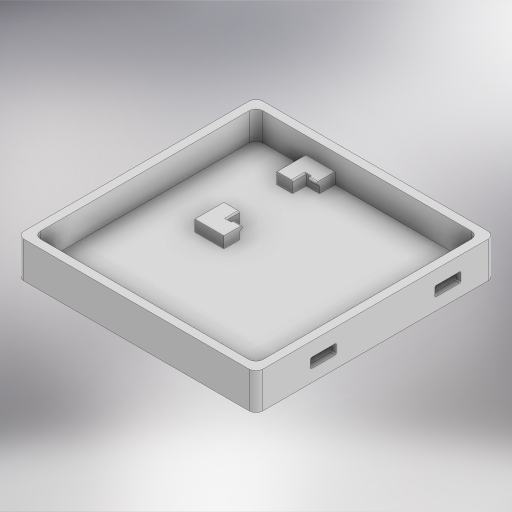
# Autodesk Inventor part: Bottom Plate
Saved by Autodesk Inventor 2024 (Build 280153000, 153)
## iProperties
Created: 2026-05-15
Part Number: Bottom Plate
Material: Generic
Document SubType Name: Modeling
Designer: Satyajit
Density: 1 g/cm^3
Appearance: Default
Author: Satyajit
Autodesk Inventor part; units mm, degrees
ref_plane "YZ Plane" through (0, 0, 0) normal (1, 0, 0) x (0, 1, 0)
ref_plane "XZ Plane" through (0, 0, 0) normal (0, 1, 0) x (-1, 0, 0)
ref_plane "XY Plane" through (0, 0, 0) normal (0, 0, 1) x (1, 0, 0)
sketch "Sketch1" plane through (0, 0, 0) normal (0, 1, 0) x (-1, 0, 0)
  line L0 (40, -40) -> (-40, -40)
  line L1 (-40, -40) -> (-40, 40)
  line L2 (-40, 40) -> (40, 40)
  line L3 (40, 40) -> (40, -40)
  line L4 (40, -40) -> (-40, 40) construction
  line L5 (-40, -40) -> (40, 40) construction
  line L6 (-43, 43) -> (-43, -43)
  line L7 (-43, -43) -> (43, -43)
  line L8 (43, -43) -> (43, 43)
  line L9 (43, 43) -> (-43, 43)
  point P0 (0, 0)
  dimension "d0" = 80
  dimension "d1" = 3
  constraints: 20 end point, 4 parallel, 3 perpendicular, 2 midpoint, 1 horizontal, 3 other
  measures "d0" distance of L1.end L2.end
  measures "d1" distance between parallel lines of L1 L6
extrude "Extrusion1" add sketch "Sketch1" against normal blind 3 contours L0 L1 L2 L3 | L9 L8 L7 L6
extrude "Extrusion2" add sketch "Sketch1" along normal blind 10
sketch "Sketch2" plane through (0, 0, 0) normal (0, 1, 0) x (1, 0, 0)
  line L0 (-16, 34) -> (41, 34)
  line L1 (41, 34) -> (41, 6)
  line L2 (41, 6) -> (-16, 6)
  line L3 (-16, 6) -> (-16, 34) construction
  line L4 (-16, 34) -> (41, 6) construction
  line L5 (41, 34) -> (-16, 6) construction
  line L6 (-16, 29.15) -> (-22, 29.15) construction
  line L7 (-22, 29.15) -> (-22, 10.85) construction
  line L8 (-22, 10.85) -> (-16, 10.85) construction
  line L9 (40, 40) -> (40, -40) projected
  line L10 (-40, -40) -> (-40, 40) construction
  line L11 (43, 43) -> (43, -43) projected
  line L12 (-40, 40) -> (40, 40) projected
  line L13 (-16.4, 29.55) -> (-16.4, 34.4)
  line L14 (-16.4, 34.4) -> (-11.55, 34.4)
  line L15 (-11.55, 34.4) -> (-11.55, 40)
  line L16 (-16.4, 29.55) -> (-22, 29.55)
  line L17 (-22, 29.55) -> (-22, 40)
  line L18 (12.5, 20) -> (-22, 20) construction
  line L19 (-16.4, 10.45) -> (-16.4, 5.6)
  line L20 (-16.4, 5.6) -> (-11.55, 5.6)
  line L21 (-11.55, 5.6) -> (-11.55, 0)
  line L22 (-16.4, 10.45) -> (-22, 10.45)
  line L23 (-22, 10.45) -> (-22, 0)
  line L24 (-22, 0) -> (-11.55, 0)
  line L25 (40, 5.5) -> (41, 5.5)
  line L26 (41, 5.5) -> (41, 6)
  line L27 (40, 34) -> (40, 34.5)
  line L28 (40, 34.5) -> (41, 34.5)
  line L29 (41, 34.5) -> (41, 34)
  point P0 (0, 0)
  point P1 (40, 6)
  dimension "d16" = 57
  dimension "d17" = 28
  dimension "d18" = 6
  dimension "d19" = 18.3
  dimension "d26" = 2
  dimension "d27" = 6
  dimension "d28" = 0.4
  dimension "d29" = 0.4
  dimension "d30" = 0.4
  dimension "d35" = 0.5
  constraints: 52 end point, 11 perpendicular, 8 point on line, 6 symmetric about line, 4 horizontal, 3 midpoint, 2 collinear, 2 parallel, 1 horizontal alignment, 1 vertical, 1 other
  measures "d16" distance of L0.start L0.end
  measures "d17" distance of L0.end L1.end
  measures "d18" distance between parallel lines of L3 L7
  measures "d19" distance of L6.end L7.end
  measures "d26" distance between parallel lines of L11 L1
  measures "d27" distance between parallel lines of L12 L0
  measures "d28" distance between parallel lines of L6 L16
  measures "d29" distance between parallel lines of L13 L3
  measures "d30" distance between parallel lines of L14 L0
  measures "d35" distance of L28.end L0.end
extrude "Extrusion3" add sketch "Sketch2" along normal blind 4 contours L12 L15 L14 L13 L16 L17 | L19 L20 L21 L24 L23 L22
extrude "Extrusion4" cut sketch "Sketch2" along normal blind 6 contours L9 L28 L29 L0 | L0 L1 L2 L9 | L2 L26 L25 L9
sketch "Sketch3" plane through (41, 0, -34.5) normal (-1, 0, 0) x (0, 0, 1)
  line L0 (29, 0) -> (0, 0) projected
  line L1 (29, 0) -> (29, 6) projected
  line L2 (29, 6) -> (0, 6) projected
  line L3 (0, 0) -> (0, 6) projected
  line L4 (4.35, 1.45) -> (12.65, 1.45)
  line L5 (13.15, 1.95) -> (13.15, 4.45)
  line L6 (12.65, 4.95) -> (4.35, 4.95)
  line L7 (3.85, 4.45) -> (3.85, 1.95)
  line L8 (3.85, 1.45) -> (13.15, 4.95) construction
  line L9 (13.15, 1.45) -> (3.85, 4.95) construction
  line L10 (14.5, 0) -> (14.5, 6) construction
  line L11 (24.65, 1.45) -> (16.35, 1.45)
  line L12 (15.85, 1.95) -> (15.85, 4.45)
  line L13 (16.35, 4.95) -> (24.65, 4.95)
  line L14 (25.15, 4.45) -> (25.15, 1.95)
  line L15 (25.15, 1.45) -> (15.85, 4.95) construction
  line L16 (15.85, 1.45) -> (25.15, 4.95) construction
  arc A0 (3.85, 1.95) -> (4.35, 1.45) centre (4.35, 1.95) ccw
  arc A1 (4.35, 4.95) -> (3.85, 4.45) centre (4.35, 4.45) ccw
  arc A2 (13.15, 4.45) -> (12.65, 4.95) centre (12.65, 4.45) ccw
  arc A3 (12.65, 1.45) -> (13.15, 1.95) centre (12.65, 1.95) ccw
  arc A4 (15.85, 1.95) -> (16.35, 1.45) centre (16.35, 1.95) ccw
  arc A5 (16.35, 4.95) -> (15.85, 4.45) centre (16.35, 4.45) ccw
  arc A6 (25.15, 4.45) -> (24.65, 4.95) centre (24.65, 4.45) ccw
  arc A7 (24.65, 1.45) -> (25.15, 1.95) centre (24.65, 1.95) ccw
  line L17 (49.1, 1.45) -> (57.4, 1.45)
  line L18 (57.9, 1.95) -> (57.9, 4.45)
  line L19 (57.4, 4.95) -> (49.1, 4.95)
  line L20 (48.6, 4.45) -> (48.6, 1.95)
  line L21 (48.6, 1.45) -> (57.9, 4.95) construction
  line L22 (57.9, 1.45) -> (48.6, 4.95) construction
  arc A8 (48.6, 1.95) -> (49.1, 1.45) centre (49.1, 1.95) ccw
  arc A9 (49.1, 4.95) -> (48.6, 4.45) centre (49.1, 4.45) ccw
  arc A10 (57.9, 4.45) -> (57.4, 4.95) centre (57.4, 4.45) ccw
  arc A11 (57.4, 1.45) -> (57.9, 1.95) centre (57.4, 1.95) ccw
  line L23 (29, 0) -> (77.5, 0)
  line L24 (77.5, -3) -> (77.5, 10) projected
  line L25 (47.25, 0) -> (47.25, 6)
  line L26 (47.25, 6) -> (59.25, 6)
  line L27 (59.25, 6) -> (59.25, 0)
  point P0 (34.5, 0)
  point P1 (8.5, 3.2)
  point P2 (20.5, 3.2)
  point P3 (20.5, 3.2)
  point P4 (53.25, 3.2)
  point P5 (53.25, 0)
  point P6 (53.25, 6)
  dimension "d36" = 9.3
  dimension "d37" = 3.5
  dimension "d40" = 12
  dimension "d41" = 3.2
  dimension "d42" = 0.5
  dimension "d45" = 9.3
  dimension "d46" = 3.5
  dimension "d47" = 0.5
  dimension "d48" = 12
  constraints: 46 end point, 27 point on line, 24 point on circle, 24 tangent, 12 centre point, 10 equal radius, 9 midpoint, 5 parallel, 5 symmetric about line, 4 perpendicular, 3 horizontal, 2 vertical alignment, 1 horizontal alignment, 1 vertical
  measures "d36" distance of L8.end L9.end
  measures "d37" distance of L9.start L8.end
  measures "d40" distance of point (8.5, 3.2) point (20.5, 3.2)
  measures "d41" distance from line of L0 point (8.5, 3.2)
  measures "d42" radius of A0
  measures "d45" distance of L21.end L22.end
  measures "d46" distance of L22.start L21.end
  measures "d47" radius of A8
  measures "d48" distance between parallel lines of L27 L25
extrude "Extrusion5" cut sketch "Sketch3" against normal blind 6 contours A0 L7 A1 L6 A2 L5 A3 L4 | A8 L20 A9 L19 A10 L18 A11 L17
extrude "Extrusion6" cut sketch "Sketch3" along normal blind 6 contours A8 L20 A9 L19 A10 L18 A11 L17 | L25 L26 L27 L23
sketch "Sketch4" plane through (0, 4, 0) normal (0, 1, 0) x (1, 0, 0)
  line L0 (-11.55, 5.6) -> (-16.4, 5.6) projected
  line L1 (-16.4, 5.6) -> (-16.4, 10.45) projected
  line L2 (-11.55, 0) -> (-11.55, 5.6) projected
  line L3 (-11.55, 5.6) -> (-11.55, 6.6)
  line L4 (-11.55, 6.6) -> (-14.55, 6.6)
  line L5 (-14.55, 6.6) -> (-14.55, 5.6)
  line L6 (-16.4, 10.45) -> (-22, 10.45) projected
  line L7 (-22, 40) -> (-22, 29.55) projected
  line L8 (-22, 10.45) -> (-22, 29.55) construction
  line L9 (-22, 20) -> (0, 20) construction
  line L10 (-22, 29.55) -> (-16.4, 29.55) projected
  line L11 (-16.4, 29.55) -> (-16.4, 34.4) projected
  line L12 (-16.4, 34.4) -> (-11.55, 34.4) projected
  line L13 (-11.55, 34.4) -> (-11.55, 33.4)
  line L14 (-11.55, 33.4) -> (-14.55, 33.4)
  line L15 (-14.55, 33.4) -> (-14.55, 34.4)
  point P0 (0, 0)
  dimension "d51" = 1
  dimension "d52" = 3
  constraints: 16 end point, 3 symmetric about line, 2 perpendicular, 2 vertical, 1 horizontal, 1 midpoint, 1 point on line, 1 vertical alignment
  measures "d51" distance of L0.start L3.end
  measures "d52" distance of L3.end L4.end
extrude "Extrusion7" add sketch "Sketch4" against normal blind 1
fillet "Fillet1" radius 0.5 4 edges at (-13.05, 4, -6.6) (-13.05, 3, -6.6) (-13.05, 4, -33.4) (-13.05, 3, -33.4)
fillet "Fillet2" radius 1 2 edges at (-13.05, 3, -5.6) (-13.05, 3, -34.4)
fillet "Fillet3" radius 0.5 24 edges at (-16.4, 4, -31.975) (-16.4, 4, -8.025) (41, 1.5964, -30.5036) (41, 3.2, -30.65) (41, 4.8036, -30.5036) (41, 4.95, -26) (41, 4.8036, -21.4964) (41, 3.2, -21.35) (41, 1.5964, -21.4964) (41, 1.45, -26) (40, 3, -34.5) (40, 6, -20) (40, 3, -5.5) (41, 1.5964, 23.2536) (41, 3.2, 23.4) (41, 4.8036, 23.2536) (41, 4.95, 18.75) (41, 4.8036, 14.2464) (41, 3.2, 14.1) (41, 1.5964, 14.2464) (41, 1.45, 18.75) (40, 3, 12.75) (40, 6, 18.75) (40, 3, 24.75)
fillet "Fillet4" radius 2.5 8 edges at (40, 5, -40) (43, 3.5, -43) (43, 3.5, 43) (40, 5, 40) (-43, 3.5, -43) (-43, 3.5, 43) (-40, 5, 40) (-40, 5, -40)
body "Solid1"
